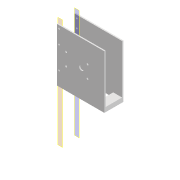
# Autodesk Inventor part: whole servo mount
Saved by Autodesk Inventor 2020 (Build 240168000, 168)
## iProperties
Created: 2019-12-15
Part Number: whole servo mount
Material: Generic
Document SubType Name: Modeling
Designer: ball
Density: 1 g/cm^3
Appearance: Default
Author: ball
Autodesk Inventor part; units mm, degrees
ref_plane "YZ Plane" through (0, 0, 0) normal (1, 0, 0) x (0, 1, 0)
ref_plane "XZ Plane" through (0, 0, 0) normal (0, 1, 0) x (-1, 0, 0)
ref_plane "XY Plane" through (0, 0, 0) normal (0, 0, 1) x (1, 0, 0)
ref_plane "Work Plane1" through (0, 0, 0) normal (0, 0, 1) x (1, 0, 0)
sketch "Sketch1" plane through (0, 0, 0) normal (0, 0, 1) x (1, 0, 0)
  circle A0 centre (4.5, -6.5) radius 1.7 construction
  circle A1 centre (4.5, -36) radius 1.7 construction
  line L0 (0, 0) -> (101.6, 0)
  line L1 (101.6, 0) -> (101.6, -114.3)
  line L2 (101.6, -114.3) -> (0, -114.3)
  line L3 (0, -114.3) -> (0, 0)
  circle A2 centre (52.3875, -55.5625) radius 4.8895
  circle A3 centre (4.5, -84) radius 1.7 construction
  circle A4 centre (4.5, -6.5) radius 1.7
  circle A5 centre (4.5, -36) radius 1.7
  circle A6 centre (4.5, -84) radius 1.7
  dimension "d0" = 101.6
  dimension "d1" = 114.3
  dimension "d2" = 9.779
  dimension "d3" = 3.4
  dimension "d4" = 3.4
  dimension "d5" = 3.4
  constraints: 8 end point, 4 centre point, 3 coincident, 2 parallel, 1 horizontal, 1 perpendicular
  measures "d0" distance of L1.end L2.end
  measures "d1" distance of L0.end L1.end
  measures "d2" diameter of A2
  measures "d3" diameter of A4
  measures "d4" diameter of A5
  measures "d5" diameter of A6
extrude "Extrusion1" add sketch "Sketch1" along normal blind 2.54
ref_plane "Work Plane2" through (0, -215, -35.5) normal (0, 0, -1) x (-1, 0, 0)
sketch "Sketch3" plane through (0, -215, -35.5) normal (0, 0, -1) x (-1, 0, 0)
  circle A0 centre (-4.5, 208.5) radius 1.7 construction
  circle A1 centre (-4.5, 189.95) radius 1.7 construction
  circle A2 centre (-4.5, 131) radius 1.7 construction
  line L0 (-101.6, 215) -> (0, 215) projected
  line L1 (0, 215) -> (-101.6, 215)
  line L2 (-101.6, 215) -> (-101.6, 100.7)
  line L3 (-101.6, 100.7) -> (0, 100.7)
  line L4 (0, 100.7) -> (0, 215)
  circle A3 centre (-52.3875, 159.4375) radius 4.8895 projected
  circle A4 centre (-4.5, 131) radius 1.7 projected
  circle A5 centre (-4.5, 131) radius 1.7
  circle A6 centre (-4.5, 189.95) radius 1.7
  circle A7 centre (-4.5, 208.5) radius 1.7 projected
  circle A8 centre (-4.5, 208.5) radius 1.7
  dimension "d13" = 114.3
  dimension "d14" = 101.6
  dimension "d15" = 3.4
  dimension "d16" = 3.4
  dimension "d17" = 3.4
  constraints: 8 end point, 3 centre point, 3 coincident, 2 parallel, 1 horizontal, 1 perpendicular
  measures "d13" distance between parallel lines of L0 L3
  measures "d14" distance between parallel lines of L4 L2
  measures "d15" diameter of A5
  measures "d16" diameter of A6
  measures "d17" diameter of A8
extrude "Extrusion2" add sketch "Sketch3" along normal blind 2.54
sketch "Sketch4" plane through (0, -215, -35.5) normal (0, 0, 1) x (1, 0, 0)
  line L0 (101.6, 100.7) -> (0, 100.7) projected
  line L1 (9.525, 100.7) -> (28.575, 100.7)
  line L2 (28.575, 100.7) -> (28.575, 110.225)
  line L3 (28.575, 110.225) -> (9.525, 110.225)
  line L4 (9.525, 110.225) -> (9.525, 100.7)
  line L5 (101.6, 100.7) -> (82.55, 100.7)
  line L6 (82.55, 100.7) -> (82.55, 110.225)
  line L7 (82.55, 110.225) -> (101.6, 110.225)
  line L8 (101.6, 110.225) -> (101.6, 100.7)
  point P0 (0, 215)
  dimension "d20" = 19.05
  dimension "d21" = 9.525
  dimension "d22" = 19.05
  dimension "d23" = 9.525
  constraints: 16 end point, 4 parallel, 2 horizontal, 2 perpendicular, 1 point on line
  measures "d20" distance of L3.end L2.end
  measures "d21" distance of L2.end L1.end
  measures "d22" distance of L6.end L7.end
  measures "d23" distance of L5.end L6.end
extrude "Extrusion3" add sketch "Sketch4" along normal up to surface (35.5 mm away)
sketch "Sketch5" plane through (0, -215, -38.04) normal (0, 0, -1) x (-1, 0, 0)
  circle A0 centre (-61.9125, 159.4375) radius 1.397
  circle A1 centre (-52.3875, 159.4375) radius 4.8895 projected
  circle A2 centre (-59.1227, 152.7023) radius 1.397
  circle A3 centre (-52.3875, 149.9125) radius 1.397
  circle A4 centre (-45.6523, 152.7023) radius 1.397
  circle A5 centre (-42.8625, 159.4375) radius 1.397
  circle A6 centre (-45.6523, 166.1727) radius 1.397
  circle A7 centre (-52.3875, 168.9625) radius 1.397
  circle A8 centre (-59.1227, 166.1727) radius 1.397
  point P0 (0, 215)
  dimension "d26" = 2.794
  dimension "d27" = 9.525
  dimension "d30" = 360
  constraints: 8 centre point, 17 other
  measures "d26" diameter of A0
  measures "d27" distance of A1.centre A0.centre
extrude "Extrusion4" cut sketch "Sketch5" against normal blind 2.54
sketch "Sketch7" plane through (0, 0, 0) normal (0, 0, -1) x (-1, 0, 0)
  circle A0 centre (-45.6523, -62.2977) radius 1.397 projected
  circle A1 centre (-45.6523, -48.8273) radius 1.397 projected
  circle A2 centre (-61.9125, -55.5625) radius 1.397 projected
  circle A3 centre (-42.8625, -55.5625) radius 1.397 projected
  circle A4 centre (-59.1227, -48.8273) radius 1.397 projected
  circle A5 centre (-59.1227, -62.2977) radius 1.397 projected
  circle A6 centre (-52.3875, -65.0875) radius 1.397 projected
  circle A7 centre (-52.3875, -46.0375) radius 1.397 projected
  line L0 (0, -114.3) -> (0, 0) projected
  line L1 (0, 0) -> (-101.6, 0) projected
  line L2 (-101.6, 0) -> (-101.6, -114.3) projected
  line L3 (-101.6, -114.3) -> (0, -114.3) projected
  circle A8 centre (-4.5, -6.5) radius 1.7 projected
  circle A9 centre (-4.5, -25.05) radius 1.7 projected
  circle A10 centre (-4.5, -84) radius 1.7 projected
  circle A11 centre (-52.3875, -55.5625) radius 4.8895 projected
  circle A12 centre (-65.5321, -42.0921) radius 1.3525 construction
  circle A13 centre (-19.5429, -42.0921) radius 1.3525 construction
  circle A14 centre (-19.5429, -69.0329) radius 1.3525 construction
  circle A15 centre (-65.5321, -69.0329) radius 1.3525 construction
  circle A16 centre (-65.5321, -69.0329) radius 1.9304
  circle A17 centre (-65.5321, -42.0921) radius 1.9304
  circle A18 centre (-19.5429, -42.0921) radius 1.9304
  circle A19 centre (-19.5429, -69.0329) radius 1.9304
  dimension "d34" = 3.8608
  dimension "d35" = 3.8608
  dimension "d36" = 3.8608
  dimension "d37" = 3.8608
  constraints: 4 centre point, 4 coincident
  measures "d34" diameter of A16
  measures "d35" diameter of A17
  measures "d36" diameter of A18
  measures "d37" diameter of A19
extrude "Extrusion5" cut sketch "Sketch7" against normal through all contours A16 | A17 | A18 | A19
equation "\"d13\" = d1"
equation "\"d14\" = d0"
body "Solid1"
